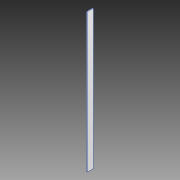
# Autodesk Inventor part: FE-130-004 End Tube Mount
Saved by Autodesk Inventor 2021 (Build 250183000, 183)
## iProperties
Created: 2021-01-11
Part Number: FE-130-004 End Tube Mount
Material: Aluminum 6061
Document SubType Name: Modeling
Density: 2.7 g/cm^3
Appearance: Aluminum - Flat
Autodesk Inventor part; units mm, degrees
ref_plane "YZ Plane" through (0, 0, 0) normal (1, 0, 0) x (0, 1, 0)
ref_plane "XZ Plane" through (0, 0, 0) normal (0, 1, 0) x (-1, 0, 0)
ref_plane "XY Plane" through (0, 0, 0) normal (0, 0, 1) x (1, 0, 0)
sketch "Sketch1" plane through (0, 0, 0) normal (1, 0, 0) x (0, 1, 0)
  line L0 (-187.325, 7.9375) -> (187.325, 7.9375)
  line L1 (187.325, 7.9375) -> (187.325, -7.9375)
  line L2 (187.325, -7.9375) -> (-187.325, -7.9375)
  line L3 (-187.325, -7.9375) -> (-187.325, 7.9375)
  line L4 (-187.325, 7.9375) -> (187.325, -7.9375) construction
  line L5 (187.325, 7.9375) -> (-187.325, -7.9375) construction
  point P0 (0, 0)
  dimension "d0" = 374.65
  dimension "d1" = 15.875
  constraints: 12 end point, 2 midpoint, 2 parallel, 1 horizontal, 1 perpendicular
  measures "d0" distance of L1.end L2.end
  measures "d1" distance of L0.end L1.end
extrude "Extrusion1" add sketch "Sketch1" along normal blind 2.3813
body "Solid1"
